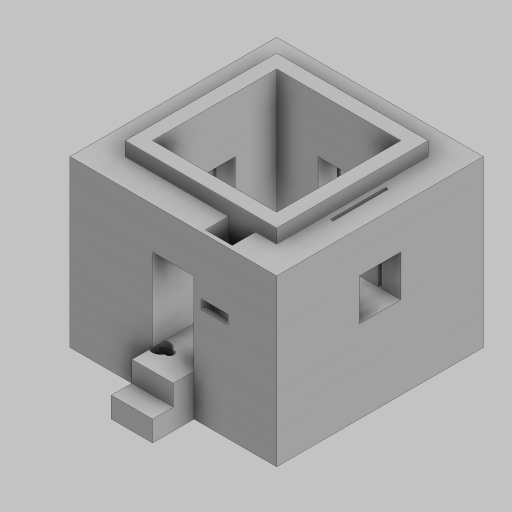
# Autodesk Inventor part: steny
Saved by Autodesk Inventor 2023 (Build 270158000, 158)
## iProperties
Created: 2022-10-19
Part Number: steny
Material: Beton
Document SubType Name: Modeling
Designer: zak
Density: 2.40731 g/cm^3
Appearance: Světle šedá
Mass: 4536.22 g
Surface Area: 1779.02 cm^2
Volume: 1884.35 cm^3
Author: zak
Autodesk Inventor part; units mm, degrees
ref_plane "YZ Plane" through (0, 0, 0) normal (1, 0, 0) x (0, 1, 0)
ref_plane "XZ Plane" through (0, 0, 0) normal (0, 1, 0) x (-1, 0, 0)
ref_plane "XY Plane" through (0, 0, 0) normal (0, 0, 1) x (1, 0, 0)
sketch "Náčrt1" plane through (0, 0, 0) normal (0, 1, 0) x (-1, 0, 0)
  line L0 (75, 75) -> (-75, 75)
  line L1 (-75, 75) -> (-75, -75)
  line L2 (-75, -75) -> (75, -75)
  line L3 (75, -75) -> (75, 75)
  line L4 (75, 75) -> (-75, -75) construction
  line L5 (-75, 75) -> (75, -75) construction
  point P0 (0, 0)
  dimension "d0" = 150
  dimension "d1" = 150
  constraints: 12 end point, 2 midpoint, 2 parallel, 1 horizontal, 1 perpendicular
  measures "d0" distance of L2.end L1.end
  measures "d1" distance of L1.end L0.end
extrude "Vysunutí1" add sketch "Náčrt1" along normal blind 30
sketch "Náčrt2" plane through (0, 30, 0) normal (0, 1, 0) x (1, 0, 0)
  line L0 (75, -75) -> (-75, -75)
  line L1 (-75, -75) -> (-75, 75)
  line L2 (-75, 75) -> (75, 75)
  line L3 (75, 75) -> (75, -75)
  line L4 (75, -75) -> (-75, 75) construction
  line L5 (-75, -75) -> (75, 75) construction
  line L6 (45, -45) -> (-45, -45)
  line L7 (-45, -45) -> (-45, 45)
  line L8 (-45, 45) -> (45, 45)
  line L9 (45, 45) -> (45, -45)
  line L10 (45, -45) -> (-45, 45) construction
  line L11 (-45, -45) -> (45, 45) construction
  point P0 (0, 0)
  dimension "d4" = 150
  dimension "d5" = 150
  dimension "d6" = 90
  dimension "d7" = 90
  constraints: 24 end point, 4 midpoint, 4 parallel, 2 horizontal, 2 perpendicular
  measures "d4" distance of L1.end L2.end
  measures "d5" distance of L0.end L1.end
  measures "d6" distance of L7.end L8.end
  measures "d7" distance of L6.end L7.end
extrude "Vysunutí2" add sketch "Náčrt2" along normal blind 90
sketch "Náčrt3" plane through (-75, 0, 75) normal (0, 0, 1) x (1, 0, 0)
  line L0 (120, 30) -> (30, 30) projected
  line L1 (60, 30) -> (90, 30)
  line L2 (90, 30) -> (90, 90)
  line L3 (90, 90) -> (60, 90)
  line L4 (60, 90) -> (60, 30)
  point P0 (75, 0)
  dimension "d10" = 30
  dimension "d11" = 60
  constraints: 8 end point, 2 parallel, 1 horizontal, 1 perpendicular, 1 point on line
  measures "d10" distance of L3.end L2.end
  measures "d11" distance of L2.end L1.end
extrude "Vysunutí3" cut sketch "Náčrt3" against normal blind 90
sketch "Náčrt4" plane through (75, 0, 75) normal (1, 0, 0) x (0, 0, -1)
  line L0 (60, 60) -> (90, 60)
  line L1 (90, 60) -> (90, 90)
  line L2 (90, 90) -> (60, 90)
  line L3 (60, 90) -> (60, 60)
  point P0 (75, 0)
  dimension "d14" = 30
  dimension "d15" = 30
  constraints: 8 end point, 2 parallel, 1 horizontal, 1 perpendicular
  measures "d14" distance of L2.end L1.end
  measures "d15" distance of L1.end L0.end
extrude "Vysunutí4" cut sketch "Náčrt4" against normal through all
sketch "Náčrt5" plane through (75, 0, -75) normal (0, 0, -1) x (-1, 0, 0)
  line L0 (60, 30) -> (60, 90) projected
  line L1 (60, 90) -> (90, 90)
  line L2 (90, 90) -> (90, 60)
  line L3 (90, 60) -> (60, 60)
  line L4 (60, 60) -> (60, 90)
  point P0 (75, 0)
  dimension "d18" = 30
  dimension "d19" = 30
  constraints: 8 end point, 2 parallel, 1 horizontal, 1 perpendicular
  measures "d18" distance of L2.end L3.end
  measures "d19" distance of L1.end L2.end
extrude "Vysunutí5" cut sketch "Náčrt5" against normal through all
sketch "Náčrt6" plane through (0, 0, 0) normal (1, 0, 0) x (0, 1, 0)
  line L0 (0, 75) -> (120, 75) projected
  line L1 (0, 75) -> (0, -75) projected
  line L2 (0, 75) -> (30, 75)
  line L3 (30, 75) -> (30, 105)
  line L4 (30, 105) -> (0, 105)
  line L5 (0, 105) -> (0, 75)
  line L6 (30, 105) -> (15, 105)
  line L7 (15, 105) -> (15, 90)
  line L8 (15, 90) -> (30, 90)
  line L9 (30, 90) -> (30, 105)
  point P0 (0, 0)
  dimension "d28" = 30
  dimension "d29" = 30
  dimension "d30" = 15
  dimension "d31" = 15
  constraints: 16 end point, 4 parallel, 2 horizontal, 2 perpendicular
  measures "d28" distance of L4.end L3.end
  measures "d29" distance of L3.end L2.end
  measures "d30" distance of L8.end L7.end
  measures "d31" distance of L7.end L6.end
extrude "Vysunutí6" add sketch "Náčrt6" along normal mid plane 30 contours L5 L4 L7 L8 L3 L0
sketch "Náčrt7" plane through (0, 120, 0) normal (0, 1, 0) x (1, 0, 0)
  line L0 (15, -45) -> (45, -45) projected
  line L1 (-45, 45) -> (45, 45)
  line L2 (45, 45) -> (45, -45)
  line L3 (45, -45) -> (-45, -45)
  line L4 (-45, -45) -> (-45, 45)
  line L5 (-45, 45) -> (45, -45) construction
  line L6 (45, 45) -> (-45, -45) construction
  line L7 (-55, 55) -> (55, 55)
  line L8 (55, 55) -> (55, -55)
  line L9 (55, -55) -> (-55, -55)
  line L10 (-55, -55) -> (-55, 55)
  line L11 (-55, 55) -> (55, -55) construction
  line L12 (55, 55) -> (-55, -55) construction
  point P0 (0, 0)
  dimension "d32" = 110
  dimension "d33" = 110
  constraints: 24 end point, 4 midpoint, 4 parallel, 2 horizontal, 2 perpendicular
  measures "d32" distance of L8.end L9.end
  measures "d33" distance of L7.end L8.end
extrude "Vysunutí7" add sketch "Náčrt7" along normal blind 10
sketch "Náčrt9" plane through (0, 0, 0) normal (0, -1, 0) x (1, 0, 0)
  line L0 (75, 75) -> (75, -75) projected
  line L1 (-75, 75) -> (-15, 75) projected
  point P0 (0, 0)
  point P1 (60, 60)
  point P2 (60, -60)
  point P3 (-60, -60)
  point P4 (-60, 60)
  dimension "d48" = 120
  dimension "d49" = 120
  dimension "d50" = 15
  dimension "d58" = 15
  constraints: 2 horizontal alignment, 2 vertical alignment
  measures "d48" distance of point (60, -60) point (60, 60)
  measures "d49" distance of point (-60, -60) point (60, -60)
  measures "d50" distance from line of L0 point (60, -60)
  measures "d58" distance from line of L1 point (-60, 60)
hole "Díra1" at (60, 0, 60) at (60, 0, -60) at (-60, 0, -60) at (-60, 0, 60) direction (0, 1, 0) diameter 10 depth 8 tip angle 118
sketch "Náčrt10" plane through (0, 120, 0) normal (0, 1, 0) x (1, 0, 0)
  line L0 (61, -20) -> (59, -20)
  line L1 (59, -20) -> (59, 20)
  line L2 (59, 20) -> (61, 20)
  line L3 (61, 20) -> (61, -20)
  line L4 (75, -75) -> (75, 75) projected
  line L5 (45, 45) -> (45, -45) projected
  line L6 (75, 15) -> (45, 15) projected
  line L7 (75, -15) -> (45, -15) projected
  line L8 (0, 17.5556) -> (0, -18.0256) construction
  line L9 (-61, -20) -> (-59, -20)
  line L10 (-59, -20) -> (-59, 20)
  line L11 (-59, 20) -> (-61, 20)
  line L12 (-61, 20) -> (-61, -20)
  line L13 (-75, 15) -> (-45, 15)
  line L14 (-75, -15) -> (-45, -15)
  line L15 (75, 75) -> (-75, 75) construction
  line L16 (0, 0) -> (-75, 75) construction
  line L17 (20, 61) -> (20, 59)
  line L18 (20, 59) -> (-20, 59)
  line L19 (-20, 59) -> (-20, 61)
  line L20 (-20, 61) -> (20, 61)
  line L21 (-15, 75) -> (-15, 45)
  line L22 (15, 75) -> (15, 45)
  point P0 (59, 0)
  point P1 (60, 20)
  point P2 (60, -20)
  point P3 (-59, 0)
  point P4 (-60, 20)
  point P5 (-60, -20)
  point P6 (0, 59)
  point P7 (-20, 60)
  point P8 (20, 60)
  dimension "d51" = 2
  dimension "d52" = 14
  dimension "d53" = 14
  dimension "d54" = 5
  dimension "d55" = 5
  constraints: 36 end point, 22 symmetric about line, 3 midpoint, 2 parallel, 1 horizontal, 1 perpendicular, 1 vertical
  measures "d51" distance from line of L3 point (59, 0)
  measures "d52" distance between parallel lines of L4 L3
  measures "d53" distance between parallel lines of L5 L1
  measures "d54" distance from line of L6 point (60, 20)
  measures "d55" distance from line of L7 point (60, -20)
extrude "Vysunutí9" cut sketch "Náčrt10" against normal blind 60 contours L0 L1 L7 L3 | L7 L1 L6 L3 | L6 L1 L2 L3 | L12 L14 L10 L9 | L12 L13 L10 L14 | L12 L11 L10 L13 | L17 L18 L22 L20 | L22 L18 L21 L20 | L21 L18 L19 L20
sketch "Náčrt11" plane through (0, 0, 0) normal (0, -1, 0) x (1, 0, 0)
  line L0 (-75, 75) -> (-15, 75) projected
  line L1 (10.5, 78.25) -> (-23.5, 78.25)
  line L2 (-23.5, 78.25) -> (-23.5, 65.75)
  line L3 (-23.5, 65.75) -> (10.5, 65.75)
  line L4 (10.5, 65.75) -> (10.5, 78.25)
  line L5 (-15, 75) -> (-15, 105) projected
  circle A0 centre (-12, 72) radius 6.25
  point P0 (0, 0)
  point P1 (-23.5, 72)
  dimension "d65" = 34
  dimension "d66" = 12.5
  dimension "d92" = 11.5
  constraints: 8 end point, 2 parallel, 1 centre point, 1 horizontal, 1 midpoint, 1 perpendicular, 1 tangent
  measures "d65" distance of L3.end L2.end
  measures "d66" distance of L2.end L1.end
  measures "d92" distance from line of L2 A0.centre
extrude "Vysunutí10" cut sketch "Náčrt11" against normal blind 21
sketch "Náčrt13" plane through (0, 21, 0) normal (0, -1, 0) x (1, 0, 0)
  line L0 (10.5, 65.75) -> (-23.5, 65.75) projected
  line L1 (-15, 78.25) -> (10.5, 78.25) projected
  line L2 (-19, 65.75) -> (5, 65.75)
  line L3 (5, 65.75) -> (5, 78.25)
  line L4 (5, 78.25) -> (-19, 78.25)
  line L5 (-19, 78.25) -> (-19, 65.75)
  line L6 (10.5, 78.25) -> (10.5, 65.75) projected
  line L7 (-23.5, 65.75) -> (-23.5, 75) projected
  point P0 (0, 0)
  point P1 (10.5, 72)
  point P2 (5, 72)
  point P3 (-19, 72)
  dimension "d79" = 24
  dimension "d80" = 5.5
  dimension "d81" = 4.5
  constraints: 8 end point, 3 midpoint, 2 parallel, 2 point on line, 1 horizontal, 1 perpendicular
  measures "d79" distance between parallel lines of L3 L5
  measures "d80" distance of point (10.5, 72) point (5, 72)
  measures "d81" distance from line of L7 point (-19, 72)
extrude "Vysunutí12" cut sketch "Náčrt13" against normal blind 4.5 contours L0 L5 L4 L1 L3
sketch "Náčrt14" plane through (0, 25.5, 0) normal (0, -1, 0) x (1, 0, 0)
  circle A0 centre (-12, 72) radius 6.25
  line L0 (-15, 78.25) -> (10.5, 78.25) projected
  line L1 (-23.5, 65.75) -> (-23.5, 75) projected
  line L2 (-19, 65.75) -> (-19, 75) projected
  circle A1 centre (-5.75, 72) radius 3
  line L3 (-15, 75) -> (-15, 78.25) projected
  point P0 (0, 0)
  point P1 (-6.47, 74.9123)
  point P2 (-6.47, 69.0877)
  dimension "d84" = 12.5
  dimension "d87" = 6
  dimension "d91" = 3
  dimension "d93" = 11.5
  constraints: 1 centre point, 1 horizontal, 3 other
  measures "d87" diameter of A1
  measures "d91" distance from line of point (-12, 72) L3
  measures "d93" distance from line of L1 point (-12, 72)
extrude "Vysunutí13" cut sketch "Náčrt14" against normal blind 4.5 contours A0 A1 | A0 A1 | A1 A0
sketch "Náčrt15" plane through (-75, 120, 75) normal (0, 0, 1) x (1, 0, 0)
  line L0 (95.25, -41.75) -> (114.75, -41.75)
  line L1 (114.75, -41.75) -> (114.75, -48.25)
  line L2 (114.75, -48.25) -> (95.25, -48.25)
  line L3 (95.25, -48.25) -> (95.25, -41.75)
  line L4 (60, -30) -> (90, -30) projected
  line L5 (90, -30) -> (120, -30)
  line L6 (120, -30) -> (120, -60)
  line L7 (120, -60) -> (90, -60)
  line L8 (90, -60) -> (90, -30)
  point P0 (75, -120)
  point P1 (105, -41.75)
  point P2 (114.75, -45)
  dimension "d95" = 30
  dimension "d96" = 6.5
  dimension "d97" = 19.5
  dimension "d98" = 15
  dimension "d99" = 15
  dimension "d100" = 15
  constraints: 16 end point, 4 parallel, 2 horizontal, 2 midpoint, 2 perpendicular
  measures "d95" distance of L6.end L7.end
  measures "d96" distance of L0.end L1.end
  measures "d97" distance between parallel lines of L1 L3
  measures "d98" distance from line of L8 point (105, -41.75)
  measures "d99" distance from line of L6 point (105, -41.75)
  measures "d100" distance from line of L5 point (114.75, -45)
extrude "Vysunutí14" cut sketch "Náčrt15" against normal blind 20 contours L0 L1 L2 L3
sketch "Náčrt16" plane through (0, 0, 0) normal (0, -1, 0) x (1, 0, 0)
  line L0 (20.25, 75) -> (20.25, 55) projected
  line L1 (39.75, 75) -> (39.75, 55) projected
  line L2 (20.25, 72) -> (39.75, 72)
  line L3 (39.75, 72) -> (39.75, 55)
  line L4 (39.75, 55) -> (20.25, 55)
  line L5 (20.25, 55) -> (20.25, 72)
  line L6 (15, 75) -> (75, 75) projected
  point P0 (0, 0)
  dimension "d103" = 17
  dimension "d104" = 3
  constraints: 8 end point, 2 parallel, 2 point on line, 1 horizontal, 1 perpendicular
  measures "d103" distance of L2.end L3.end
  measures "d104" distance between parallel lines of L6 L2
extrude "Vysunutí15" cut sketch "Náčrt16" against normal through all contours L2 L1 L4 L0
